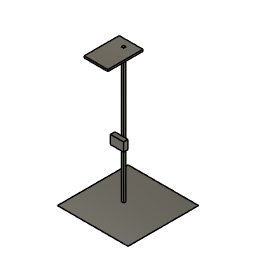
SimpleFarmer v1 (Autodesk Fusion 360 design; units mm, degrees)
Autodesk Fusion 360 part; units mm, degrees
box "BoxPrimitive2" add length 25 width 25 height 2500 placed x (0, -1, 0) y (1, 0, 0) z (0, 0, 1) at (25, 25, 0) makes body 1
box "BoxPrimitive3" add length 100 width 150 height -50 placed x (0, 0, -1) y (-1, 0, 0) z (0, 1, 0) at (100, 0, 650) separate body makes body 2
box "BoxPrimitive4" add length 800 width 800 height 1 placed x (0, -1, 0) y (1, 0, 0) z (0, 0, 1) at (-300, 400, 0) separate body makes body 3
move_body "Move1" bodies 3 to x (1, 0, 0) y (0, 1, 0) z (0, 0, 1) at (0, 0, 2500)
move_body "Move2" bodies 3 to x (1, 0, 0) y (0, 1, 0) z (0, 0, 1) at (0, 0, -2500)
box "BoxPrimitive5" add length 398.111 width 269.302 height 20 placed x (0, -1, 0) y (1, 0, 0) z (0, 0, 1) at (-700, 100, 0) separate body makes body 4
move_body "Move3" bodies 4 to x (1, 0, 0) y (0, 1, 0) z (0, 0, 1) at (600, 0, 1500)
box "BoxPrimitive6" cut length 977.112 width 498.682 height 50 placed x (0, 0, -1) y (-1, 0, 0) z (0, 1, 0) at (275.7297, 0, 2501.8992) bodies 1
